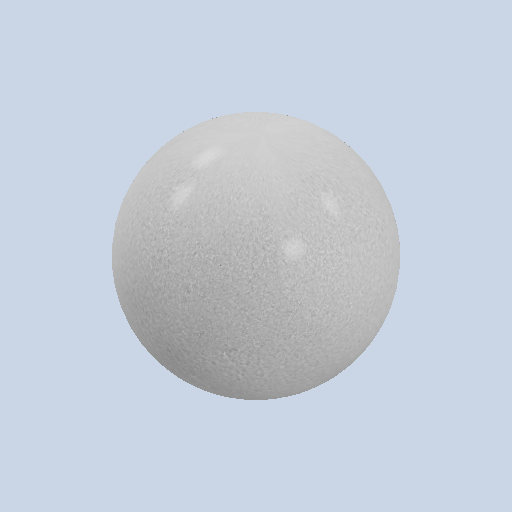
# Autodesk Inventor part: Ball
Saved by Autodesk Inventor 2023 (Build 270158000, 158)
## iProperties
Created: 2022-07-11
Part Number: Ball
Material: GFRC
Document SubType Name: Modeling
Designer: Pratyush
Density: 1.7 g/cm^3
Appearance: Flat - Polished Gray
Author: Pratyush
Autodesk Inventor part; units mm, degrees
ref_plane "YZ Plane" through (0, 0, 0) normal (1, 0, 0) x (0, 1, 0)
ref_plane "XZ Plane" through (0, 0, 0) normal (0, 1, 0) x (-1, 0, 0)
ref_plane "XY Plane" through (0, 0, 0) normal (0, 0, 1) x (1, 0, 0)
sketch "Sketch1" plane through (0, 0, 0) normal (0, 1, 0) x (-1, 0, 0)
  circle A0 centre (0, 0) radius 114.3
  dimension "d0" = 228.6
  constraints: 1 centre point, 1 coincident
  measures "d0" diameter of A0
extrude "Extrusion1" add sketch "Sketch1" along normal mid plane 228.6
fillet "Fillet1" radius 114.3 1 edges at (114.3, 114.3, 0)
fillet "Fillet2" radius 114.3 1 edges at (114.3, -114.3, 0)
body "Solid1"
